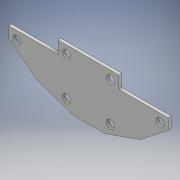
# Autodesk Inventor part: Keyboard1
Saved by Autodesk Inventor 2017 (Build 210142000, 142)
## iProperties
Created: 2017-04-18
Part Number: Keyboard1
Material: Generic
Document SubType Name: Modeling
Designer: Oleg
Density: 1 g/cm^3
Appearance: Default
Author: Oleg
Autodesk Inventor part; units mm, degrees
ref_plane "YZ Plane" through (0, 0, 0) normal (1, 0, 0) x (0, 1, 0)
ref_plane "XZ Plane" through (0, 0, 0) normal (0, 1, 0) x (-1, 0, 0)
ref_plane "XY Plane" through (0, 0, 0) normal (0, 0, 1) x (1, 0, 0)
sketch "Sketch1" plane through (0, 0, 0) normal (0, 1, 0) x (-1, 0, 0)
  circle A0 centre (48.634, 12.202) radius 1.778
  line L0 (26.207, 8.6831) -> (32.8491, 8.6831)
  line L1 (32.8491, 8.6831) -> (32.8491, 2.549)
  line L2 (32.8491, 2.549) -> (26.207, 2.549)
  line L3 (26.207, 2.549) -> (26.207, 8.6831)
  circle A1 centre (29.509, 5.597) radius 1.778
  circle A2 centre (37, 18) radius 1.5
  circle A3 centre (21, 18) radius 1.5
  circle A4 centre (3, 13.5) radius 1.5
  line L4 (32.7471, 9.6911) -> (26.105, 9.6911)
  circle A5 centre (21, 4) radius 1.5
  circle A6 centre (37, 4) radius 1.5
  circle A7 centre (55, 13.5) radius 1.5
  line L5 (8.337, 15.4121) -> (14.9791, 15.4121)
  line L6 (14.9791, 15.4121) -> (14.9791, 9.3161)
  line L7 (14.9791, 9.3161) -> (8.337, 9.3161)
  line L8 (8.337, 9.3161) -> (8.337, 15.4121)
  circle A8 centre (11.639, 12.326) radius 1.778
  line L9 (17.3531, 14.417) -> (23.4491, 14.417)
  line L10 (23.4491, 14.417) -> (23.4491, 7.7749)
  line L11 (23.4491, 7.7749) -> (17.3531, 7.7749)
  line L12 (17.3531, 7.7749) -> (17.3531, 14.417)
  circle A9 centre (20.363, 11.115) radius 1.778
  line L13 (26.105, 15.7871) -> (32.7471, 15.7871)
  line L14 (32.7471, 15.7871) -> (32.7471, 9.6911)
  line L15 (26.105, 9.6911) -> (26.105, 15.7871)
  circle A10 centre (29.407, 12.701) radius 1.778
  circle A11 centre (38.211, 11.232) radius 1.778
  line L16 (35.2011, 14.534) -> (41.259, 14.534)
  line L17 (41.259, 14.534) -> (41.259, 7.93)
  line L18 (41.259, 7.93) -> (35.2011, 7.93)
  line L19 (35.2011, 7.93) -> (35.2011, 14.534)
  line L20 (45.332, 15.2119) -> (51.9741, 15.2119)
  line L21 (51.9741, 15.2119) -> (51.9741, 9.1159)
  line L22 (51.9741, 9.1159) -> (45.332, 9.1159)
  line L23 (45.332, 9.1159) -> (45.332, 15.2119)
  line L24 (10.2856, 4.4998) -> (-0.0002, 12.5003)
  line L25 (34.6899, 0.0005) -> (47.7142, 4.5002)
  line L26 (57.9997, 16.5) -> (40.0003, 16.5)
  line L27 (39.9997, 21) -> (17.9997, 21)
  line L28 (-0.0003, 16.5) -> (18.0003, 16.5)
  line L29 (10.2856, 4.4998) -> (23.0001, 0.0002)
  line L30 (47.7142, 4.5002) -> (57.9998, 12.5002)
  line L31 (57.9997, 16.5) -> (57.9998, 12.5002)
  line L32 (34.6899, 0.0005) -> (23.0001, 0.0002)
  line L33 (-0.0002, 12.5003) -> (-0.0003, 16.5)
  line L34 (18.0003, 16.5) -> (17.9997, 21)
  line L35 (39.9997, 21) -> (40.0003, 16.5)
  point P0 (0, 0)
  constraints: 72 end point, 14 horizontal, 12 centre point, 12 vertical, 2 parallel, 2 perpendicular, 83 other
extrude "Extrusion1" add sketch "Sketch1" along normal blind 1 contours A0 | L0 L1 L2 L3 | A1 | L4 L15 L13 L14 | L5 L6 L7 L8 | A8 | L9 L10 L11 L12 | A9 | A10 | A11 | L16 L17 L18 L19 | L20 L21 L22 L23 | L24 L33 L28 L34 L27 L35 L26 L31 L30 L25 L32 L29
body "Solid1"
